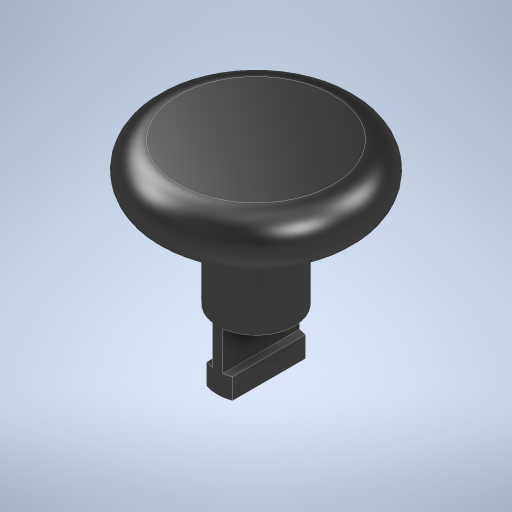
# Autodesk Inventor part: Taster_Top
Saved by Autodesk Inventor 2023.1 (Build 271208000, 208)
## iProperties
Created: 2023-12-10
Part Number: Taster_Top
Material: Generisch
Document SubType Name: Modeling
Designer: JansenL
Density: 1 g/cm^3
Appearance: Glossy - Black
Author: JansenL
Autodesk Inventor part; units mm, degrees
ref_plane "YZ Plane" through (0, 0, 0) normal (1, 0, 0) x (0, 1, 0)
ref_plane "XZ Plane" through (0, 0, 0) normal (0, 1, 0) x (-1, 0, 0)
ref_plane "XY Plane" through (0, 0, 0) normal (0, 0, 1) x (1, 0, 0)
sketch "Sketch1" plane through (0, 0, 0) normal (0, 0, 1) x (1, 0, 0)
  line L0 (-0.2, 0.9842) -> (-0.2, 0.8)
  line L1 (-0.2, 0.8) -> (-0.5, 0.8)
  line L2 (-0.5, 0.8) -> (-0.5, 0)
  line L3 (-0.5, 0) -> (0.5, 0)
  line L4 (0.5, 0) -> (0.5, 0.8)
  line L5 (0.5, 0.8) -> (0.2, 0.8)
  line L6 (0.2, 0.8) -> (0.2, 0.9842)
  line L7 (0.2, 0.9842) -> (0.2, 2.3)
  line L8 (0.2, 2.3) -> (1.5, 2.3)
  line L9 (1.5, 2.3) -> (1.5, 5.8)
  line L10 (1.5, 5.8) -> (-1.5, 5.8)
  line L11 (-1.5, 5.8) -> (-1.5, 2.3)
  line L12 (-1.5, 2.3) -> (-0.2, 2.3)
  line L13 (-0.2, 0.9842) -> (-0.2, 2.3)
  line L14 (0, 5.8) -> (0, 0) construction
  line L15 (-0.2, 2.3) -> (0.2, 2.3)
  line L16 (0, 5.8) -> (0, 2.3)
  line L17 (0, 5.8) -> (3, 5.8)
  line L18 (4, 6.8) -> (4, 6.8)
  line L19 (3, 7.8) -> (0, 7.8)
  line L20 (0, 7.8) -> (0, 5.8)
  arc A0 (4, 6.8) -> (3, 7.8) centre (3, 6.8) ccw
  arc A1 (3, 5.8) -> (4, 6.8) centre (3, 6.8) ccw
  point P0 (4, 7.8)
  point P1 (4, 5.8)
  point P2 (4, 6.8)
  dimension "d0" = 0.4
  dimension "d1" = 3
  dimension "d2" = 1
  dimension "d3" = 0.8
  dimension "d4" = 1.5
  dimension "d5" = 3.5
  dimension "d12" = 2
  dimension "d13" = 1
  dimension "d14" = 1
  dimension "d15" = 3
  constraints: 42 end point, 11 perpendicular, 10 point on line, 4 point on circle, 4 tangent, 3 midpoint, 2 centre point, 2 horizontal, 2 parallel, 2 vertical, 1 coincident, 1 other
  measures "d0" distance between parallel lines of L7 L13
  measures "d1" distance of L9.end L10.end
  measures "d2" distance of L2.end L3.end
  measures "d3" distance of L1.end L2.end
  measures "d4" distance between parallel lines of L1 L12
  measures "d5" distance of L10.end L11.end
  measures "d12" distance of point (4, 5.8) point (4, 7.8)
  measures "d13" radius of A0
  measures "d14" radius of A1
  measures "d15" distance from line of L20 A0.centre
extrude "Extrusion1" add sketch "Sketch1" along normal mid plane 3 contours L13 L15 L7 L6 L5 L4 L3 L2 L1 L0
revolve "Revolution1" add sketch "Sketch1" angle 360 about axis through (0, 5.8, 0) along (0, -1, 0) contours L16 L10 L9 L8 L15
sketch "Sketch2" plane through (-0.5, 0, 1.5) normal (0, -1, 0) x (1, 0, 0)
  circle A0 centre (0.5, -1.5) radius 1.5
  arc A1 (0.3, -0.0134) -> (0.3, -2.9866) centre (0.5, -1.5) ccw projected
  line L0 (0, -0.0858) -> (0, 0)
  line L1 (0, 0) -> (0.5, 0)
  line L2 (0, 0) -> (1, 0) projected
  line L3 (1, 0) -> (0.7, 0) projected
  line L4 (0.5, 0) -> (1, 0)
  line L5 (1, 0) -> (1, -0.0858)
  line L6 (0, -3) -> (0, 0) projected
  line L7 (0, -2.9142) -> (0, -3)
  line L8 (0.3, -3) -> (0.5, -3) projected
  line L9 (0, -3) -> (0.5, -3)
  line L10 (1, -3) -> (1, 0) projected
  line L11 (0.5, -3) -> (1, -3)
  line L12 (1, -3) -> (1, -2.9142)
  dimension "d9" = 3
  constraints: 16 end point, 6 collinear, 4 point on circle, 2 point on line, 1 centre point, 1 coincident, 1 horizontal, 1 midpoint, 1 vertical
  measures "d9" diameter of A0
extrude "Extrusion2" cut sketch "Sketch2" against normal up to surface (2.3 mm away) contours A0 L2 L5 | L10 L11 A0 | A0 L0 L1 | L8 L9 L6 A0
revolve "Revolution2" add sketch "Sketch1" angle 360 about axis through (0, 7.8, 0) along (0, -1, 0) contours L20 L19 A0 A1 L17 L10
body "Solid1"
